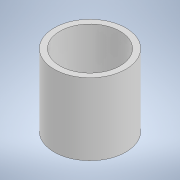
# Autodesk Inventor part: Cylinder_500ml
Saved by Autodesk Inventor 2020 (Build 240168000, 168)
## iProperties
Created: 2023-05-12
Part Number: Cylinder_500ml
Material: Generic
Document SubType Name: Modeling
Designer: DSOB
Density: 1 g/cm^3
Appearance: Default
Author: DSOB
Autodesk Inventor part; units mm, degrees
ref_plane "YZ Plane" through (0, 0, 0) normal (1, 0, 0) x (0, 1, 0)
ref_plane "XZ Plane" through (0, 0, 0) normal (0, 1, 0) x (-1, 0, 0)
ref_plane "XY Plane" through (0, 0, 0) normal (0, 0, 1) x (1, 0, 0)
sketch "Sketch1" plane through (0, 0, 0) normal (0, 1, 0) x (-1, 0, 0)
  circle A0 centre (0, 0) radius 50
  dimension "d0" = 100
  constraints: 1 centre point, 1 coincident
  measures "d0" diameter of A0
extrude "Extrusion1" add sketch "Sketch1" along normal blind 10
sketch "Sketch2" plane through (0, 10, 0) normal (0, 1, 0) x (1, 0, 0)
  circle A0 centre (0, 0) radius 50
  circle A1 centre (0, 0) radius 42
  dimension "d3" = 84
  dimension "d4" = 100
  constraints: 2 centre point, 2 coincident
  measures "d3" diameter of A1
  measures "d4" diameter of A0
extrude "Extrusion2" add sketch "Sketch2" along normal blind 90.2239
body "Solid1"
